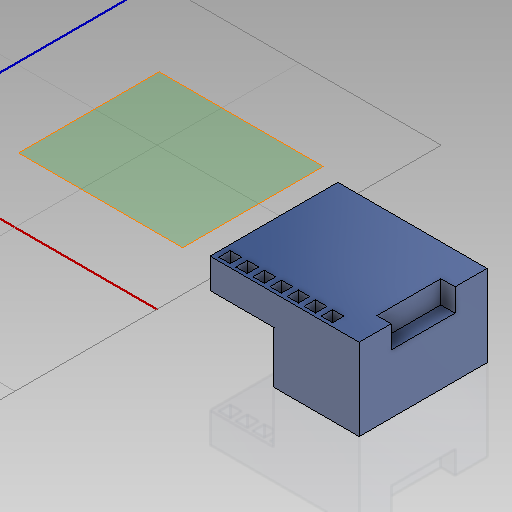
# Autodesk Inventor part: ЛЦМК0000002.00.00.00.00.04
Saved by Autodesk Inventor 2021.2 (Build 252289000, 289)
## iProperties
Created: 2025-10-23
Part Number: ЛЦМК0000002.00.00.00.00.04
Material: Типовые
Document SubType Name: Modeling
Designer: Захаров
Density: 1 g/cm^3
Appearance: С вкраплениями — сатинированная — синяя
Author: Захаров
Autodesk Inventor part; units mm, degrees
ref_plane "YZ Plane" through (0, 0, 0) normal (1, 0, 0) x (0, 1, 0)
ref_plane "XZ Plane" through (0, 0, 0) normal (0, 1, 0) x (-1, 0, 0)
ref_plane "XY Plane" through (0, 0, 0) normal (0, 0, 1) x (1, 0, 0)
ref_plane "РабПлоскость1" through (34.25, -2.8, -7.7) normal (0, -1, 0) x (1, 0, 0)
sketch "Эскиз1" plane through (34.25, -2.8, -7.7) normal (0, -1, 0) x (1, 0, 0)
  line L0 (21.65, 6.9) -> (20.05, 6.9) projected
  line L1 (20.05, 6.9) -> (20.05, 8.5) projected
  line L2 (20.05, 8.5) -> (21.65, 8.5) projected
  line L3 (21.65, 8.5) -> (21.65, 6.9) projected
  line L4 (16.85, 6.9) -> (15.25, 6.9) projected
  line L5 (15.25, 6.9) -> (15.25, 8.5) projected
  line L6 (15.25, 8.5) -> (16.85, 8.5) projected
  line L7 (16.85, 8.5) -> (16.85, 6.9) projected
  line L8 (26.45, 6.9) -> (24.85, 6.9) projected
  line L9 (24.85, 6.9) -> (24.85, 8.5) projected
  line L10 (24.85, 8.5) -> (26.45, 8.5) projected
  line L11 (26.45, 8.5) -> (26.45, 6.9) projected
  line L12 (24.05, 6.9) -> (22.45, 6.9) projected
  line L13 (22.45, 6.9) -> (22.45, 8.5) projected
  line L14 (22.45, 8.5) -> (24.05, 8.5) projected
  line L15 (24.05, 8.5) -> (24.05, 6.9) projected
  line L16 (28.85, 6.9) -> (27.25, 6.9) projected
  line L17 (27.25, 6.9) -> (27.25, 8.5) projected
  line L18 (27.25, 8.5) -> (28.85, 8.5) projected
  line L19 (28.85, 8.5) -> (28.85, 6.9) projected
  line L20 (19.25, 6.9) -> (17.65, 6.9) projected
  line L21 (17.65, 6.9) -> (17.65, 8.5) projected
  line L22 (17.65, 8.5) -> (19.25, 8.5) projected
  line L23 (19.25, 8.5) -> (19.25, 6.9) projected
  line L24 (31.25, 6.9) -> (29.65, 6.9) projected
  line L25 (29.65, 6.9) -> (29.65, 8.5) projected
  line L26 (29.65, 8.5) -> (31.25, 8.5) projected
  line L27 (31.25, 8.5) -> (31.25, 6.9) projected
  line L28 (33.5, 4.5) -> (35.5, 4.5) projected
  line L29 (35.5, 4.5) -> (35.5, 9) projected
  line L30 (35.5, 9) -> (14.5, 9) projected
  line L31 (14.5, 9) -> (14.5, -9) projected
  line L32 (14.5, -9) -> (35.5, -9) projected
  line L33 (35.5, -9) -> (35.5, -4.5) projected
  line L34 (35.5, -4.5) -> (33.5, -4.5) projected
  line L35 (33.5, -4.5) -> (33.5, 4.5) projected
  line L36 (20.05, -6.9) -> (21.65, -6.9) projected
  line L37 (21.65, -6.9) -> (21.65, -8.5) projected
  line L38 (21.65, -8.5) -> (20.05, -8.5) projected
  line L39 (20.05, -8.5) -> (20.05, -6.9) projected
  line L40 (15.25, -6.9) -> (16.85, -6.9) projected
  line L41 (16.85, -6.9) -> (16.85, -8.5) projected
  line L42 (16.85, -8.5) -> (15.25, -8.5) projected
  line L43 (15.25, -8.5) -> (15.25, -6.9) projected
  line L44 (24.85, -6.9) -> (26.45, -6.9) projected
  line L45 (26.45, -6.9) -> (26.45, -8.5) projected
  line L46 (26.45, -8.5) -> (24.85, -8.5) projected
  line L47 (24.85, -8.5) -> (24.85, -6.9) projected
  line L48 (22.45, -6.9) -> (24.05, -6.9) projected
  line L49 (24.05, -6.9) -> (24.05, -8.5) projected
  line L50 (24.05, -8.5) -> (22.45, -8.5) projected
  line L51 (22.45, -8.5) -> (22.45, -6.9) projected
  line L52 (27.25, -6.9) -> (28.85, -6.9) projected
  line L53 (28.85, -6.9) -> (28.85, -8.5) projected
  line L54 (28.85, -8.5) -> (27.25, -8.5) projected
  line L55 (27.25, -8.5) -> (27.25, -6.9) projected
  line L56 (17.65, -6.9) -> (19.25, -6.9) projected
  line L57 (19.25, -6.9) -> (19.25, -8.5) projected
  line L58 (19.25, -8.5) -> (17.65, -8.5) projected
  line L59 (17.65, -8.5) -> (17.65, -6.9) projected
  line L60 (29.65, -6.9) -> (31.25, -6.9) projected
  line L61 (31.25, -6.9) -> (31.25, -8.5) projected
  line L62 (31.25, -8.5) -> (29.65, -8.5) projected
  line L63 (29.65, -8.5) -> (29.65, -6.9) projected
  point P0 (-34.25, 7.7)
extrude "Выдавливание1" add sketch "Эскиз1" along normal blind 4.2 contours L35 L34 L33 L32 L31 L30 L29 L28 | L36 L37 L38 L39 | L40 L41 L42 L43 | L44 L45 L46 L47 | L48 L49 L50 L51 | L52 L53 L54 L55 | L56 L57 L58 L59 | L60 L61 L62 L63
sketch "Эскиз2" plane through (34.25, -7, -7.7) normal (0, -1, 0) x (1, 0, 0)
  line L0 (35.5, -9) -> (35.5, -4.5) projected
  line L1 (35.5, 9) -> (14.5, 9) projected
  line L2 (35.5, -9) -> (23.5, -9)
  line L3 (23.5, -9) -> (23.5, 9)
  line L4 (23.5, 9) -> (35.5, 9)
  line L5 (35.5, 9) -> (35.5, -9)
  point P0 (-34.25, 7.7)
  point P1 (35.5, -4.5)
  point P2 (35.5, 9)
  dimension "d2" = 12
  constraints: 8 end point, 2 parallel, 1 horizontal, 1 perpendicular, 1 point on line
  measures "d2" distance of L3.end L4.end
extrude "Выдавливание2" add sketch "Эскиз2" along normal blind 7.3
sketch "Эскиз3" plane through (34.25, -14.3, -7.7) normal (0, -1, 0) x (1, 0, 0)
  line L0 (20.05, 6.9) -> (21.65, 6.9) projected
  line L1 (21.65, 6.9) -> (21.65, 8.5) projected
  line L2 (21.65, 8.5) -> (20.05, 8.5) projected
  line L3 (20.05, 8.5) -> (20.05, 6.9) projected
  line L4 (15.25, 6.9) -> (16.85, 6.9) projected
  line L5 (16.85, 6.9) -> (16.85, 8.5) projected
  line L6 (16.85, 8.5) -> (15.25, 8.5) projected
  line L7 (15.25, 8.5) -> (15.25, 6.9) projected
  line L8 (24.85, 6.9) -> (26.45, 6.9) projected
  line L9 (26.45, 6.9) -> (26.45, 8.5) projected
  line L10 (26.45, 8.5) -> (24.85, 8.5) projected
  line L11 (24.85, 8.5) -> (24.85, 6.9) projected
  line L12 (22.45, 6.9) -> (24.05, 6.9) projected
  line L13 (24.05, 6.9) -> (24.05, 8.5) projected
  line L14 (24.05, 8.5) -> (22.45, 8.5) projected
  line L15 (22.45, 8.5) -> (22.45, 6.9) projected
  line L16 (27.25, 6.9) -> (28.85, 6.9) projected
  line L17 (28.85, 6.9) -> (28.85, 8.5) projected
  line L18 (28.85, 8.5) -> (27.25, 8.5) projected
  line L19 (27.25, 8.5) -> (27.25, 6.9) projected
  line L20 (17.65, 6.9) -> (19.25, 6.9) projected
  line L21 (19.25, 6.9) -> (19.25, 8.5) projected
  line L22 (19.25, 8.5) -> (17.65, 8.5) projected
  line L23 (17.65, 8.5) -> (17.65, 6.9) projected
  line L24 (29.65, 6.9) -> (31.25, 6.9) projected
  line L25 (31.25, 6.9) -> (31.25, 8.5) projected
  line L26 (31.25, 8.5) -> (29.65, 8.5) projected
  line L27 (29.65, 8.5) -> (29.65, 6.9) projected
  line L28 (35.5, 9) -> (14.5, 9) projected
  line L29 (35.5, -9) -> (35.5, 9) projected
  line L30 (14.5, -9) -> (35.5, -9) projected
  line L31 (14.5, 9) -> (14.5, -9) projected
  line L32 (21.65, -6.9) -> (20.05, -6.9) projected
  line L33 (20.05, -6.9) -> (20.05, -8.5) projected
  line L34 (20.05, -8.5) -> (21.65, -8.5) projected
  line L35 (21.65, -8.5) -> (21.65, -6.9) projected
  line L36 (16.85, -6.9) -> (15.25, -6.9) projected
  line L37 (15.25, -6.9) -> (15.25, -8.5) projected
  line L38 (15.25, -8.5) -> (16.85, -8.5) projected
  line L39 (16.85, -8.5) -> (16.85, -6.9) projected
  line L40 (26.45, -6.9) -> (24.85, -6.9) projected
  line L41 (24.85, -6.9) -> (24.85, -8.5) projected
  line L42 (24.85, -8.5) -> (26.45, -8.5) projected
  line L43 (26.45, -8.5) -> (26.45, -6.9) projected
  line L44 (24.05, -6.9) -> (22.45, -6.9) projected
  line L45 (22.45, -6.9) -> (22.45, -8.5) projected
  line L46 (22.45, -8.5) -> (24.05, -8.5) projected
  line L47 (24.05, -8.5) -> (24.05, -6.9) projected
  line L48 (28.85, -6.9) -> (27.25, -6.9) projected
  line L49 (27.25, -6.9) -> (27.25, -8.5) projected
  line L50 (27.25, -8.5) -> (28.85, -8.5) projected
  line L51 (28.85, -8.5) -> (28.85, -6.9) projected
  line L52 (19.25, -6.9) -> (17.65, -6.9) projected
  line L53 (17.65, -6.9) -> (17.65, -8.5) projected
  line L54 (17.65, -8.5) -> (19.25, -8.5) projected
  line L55 (19.25, -8.5) -> (19.25, -6.9) projected
  line L56 (31.25, -6.9) -> (29.65, -6.9) projected
  line L57 (29.65, -6.9) -> (29.65, -8.5) projected
  line L58 (29.65, -8.5) -> (31.25, -8.5) projected
  line L59 (31.25, -8.5) -> (31.25, -6.9) projected
  point P0 (-34.25, 7.7)
extrude "Выдавливание3" cut sketch "Эскиз3" against normal blind 7.3 contours L11 L10 L9 L8 | L15 L14 L13 L12 | L19 L18 L17 L16 | L27 L26 L25 L24
sketch "Эскиз4" plane through (34.25, -7, -7.7) normal (0, 1, 0) x (1, 0, 0)
  line L0 (33.5, -4.5) -> (35.5, -4.5) projected
  line L1 (35.5, 4.5) -> (35.5, -4.5) projected
  line L2 (35.5, 4.5) -> (33.5, 4.5) projected
  line L3 (33.5, 4.5) -> (33.5, -4.5) projected
  point P0 (-34.25, -7.7)
ref_plane "РабПлоскость2" through (10.25, -6, -12.2) normal (0, -1, 0) x (1, 0, 0)
extrude "Выдавливание4" add sketch "Эскиз4" along normal up to surface (1 mm away)
